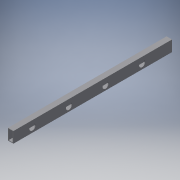
# Autodesk Inventor part: 28 Alum Tube
Saved by Autodesk Inventor 2018.2 (Build 222227000, 227)
## iProperties
Created: 2018-01-13
Part Number: 28 Alum Tube
Material: Generic
Document SubType Name: Modeling
Designer: Orangeracer
Density: 1 g/cm^3
Appearance: Default
Author: Orangeracer
Autodesk Inventor part; units mm, degrees
ref_plane "YZ Plane" through (0, 0, 0) normal (1, 0, 0) x (0, 1, 0)
ref_plane "XZ Plane" through (0, 0, 0) normal (0, 1, 0) x (-1, 0, 0)
ref_plane "XY Plane" through (0, 0, 0) normal (0, 0, 1) x (1, 0, 0)
sketch "Sketch1" plane through (0, 0, 0) normal (0, 0, 1) x (1, 0, 0)
  line L0 (0, 0) -> (-25.4, 0)
  line L1 (-25.4, 0) -> (-25.4, 50.8)
  line L2 (-25.4, 50.8) -> (0, 50.8)
  line L3 (0, 50.8) -> (0, 0)
  line L4 (-22.225, 3.175) -> (-3.175, 3.175)
  line L5 (-3.175, 3.175) -> (-3.175, 47.625)
  line L6 (-3.175, 47.625) -> (-22.225, 47.625)
  line L7 (-22.225, 47.625) -> (-22.225, 3.175)
  dimension "d0" = 25.4
  dimension "d1" = 50.8
  dimension "d2" = 3.175
  constraints: 16 end point, 4 parallel, 2 perpendicular, 1 horizontal, 3 other
  measures "d0" distance of L1.end L2.end
  measures "d1" distance of L0.end L1.end
  measures "d2" distance between parallel lines of L0 L4
extrude "Extrusion1" add sketch "Sketch1" along normal blind 736.6
sketch "Sketch2" plane through (0, 0, 0) normal (1, 0, 0) x (0, 0, -1)
  circle A0 centre (-648.589, 22.86) radius 14.2875
  circle A1 centre (-478.6704, 21.2725) radius 14.2875
  circle A2 centre (-308.7444, 21.2725) radius 14.2875
  circle A3 centre (-138.8258, 22.86) radius 14.2875
  line L0 (0, 0) -> (-736.6, 0) projected
  line L1 (-736.6, 0) -> (-736.6, 50.8) projected
  line L2 (0, 50.8) -> (0, 0) projected
  dimension "d5" = 22.86
  dimension "d6" = 21.2725
  dimension "d7" = 21.2725
  dimension "d8" = 22.86
  dimension "d9" = 169.926
  dimension "d10" = 169.926
  dimension "d11" = 169.926
  dimension "d12" = 28.575
  dimension "d13" = 28.575
  dimension "d14" = 28.575
  dimension "d15" = 28.575
  dimension "d16" = 88.011
  dimension "d17" = 138.8258
  constraints: 4 centre point
  measures "d5" distance from line of L0 A0.centre
  measures "d6" distance from line of L0 A1.centre
  measures "d7" distance from line of L0 A2.centre
  measures "d8" distance from line of L0 A3.centre
  measures "d9" distance of A1.centre A0.centre
  measures "d10" distance of A2.centre A1.centre
  measures "d11" distance of A2.centre A3.centre
  measures "d12" diameter of A0
  measures "d13" diameter of A1
  measures "d14" diameter of A2
  measures "d15" diameter of A3
  measures "d16" distance from line of L1 A0.centre
  measures "d17" distance from line of L2 A3.centre
extrude "Extrusion2" cut sketch "Sketch2" against normal blind 25.4
body "Solid1"
